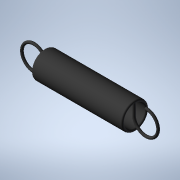
# Autodesk Inventor part: AUA2-10
Saved by Autodesk Inventor 2021 (Build 250183000, 183)
## iProperties
Created: 2025-12-16
Part Number: AUA2-10
Material: Generic
Catalog Web Link: www.3dfindit.com
Description: AWA ,AUA  ,AWY, BWY, AUY, BUY, AWU, BWU, AUU, BUU, AWS, BWS, AUS, BUSS, AWF, AUF,  AWT, BWT, AUT, BUT-Tension Springs - Extralight / Light / Light to Medium / Medium Load / Medium to Heavy / Heavy Load Type
Vendor: MISUMI
Document SubType Name: Modeling
Designer: psAdmin
Manufacturer: MISUMI
Mass: 0.00796164 g
Surface Area: 0.845602 cm^2
Volume: 0.00796164 cm^3
Density: 1 g/cm^3
Appearance: PSOLRGB-176-176-176
Category: PARTsolutions
Company: MISUMI
Title: AUA2-10
Author: Cadenas PARTsolutions
Comments: Tension Springs - Extralight / Light / Light to Medium / Medium Load / Medium to Heavy / Heavy Load Type
PSOL_IDENT_0: {$CADENAS_DATA/23d-libs/misumi/metric/29_springs/awf.prj},261 {VTYP=3D},{NB=AUA2-10},{LINA=AUA2-10},
PSOL_IDENT_1: {NN=AWA ,AUA  ,AWY, BWY, AUY, BUY, AWU, BWU, AUU, BUU, AWS, BWS, AUS, BUSS, AWF, AUF,  AWT, BWT, AUT
PSOL_IDENT_2: , BUT},{DATE=15.09.2021 11:46:20},{GEOMDATE=29.07.2021 01:15:23},{VERSION=},{LINEID=30},{WBVAR=TS,MA
PSOL_IDENT_3: T,TE,L},{WBNUMERIC=L}  {NB=AUA2-10},{LINA=AUA2-10},{KT=DUMMY},{PN=AUA2-10},{TS=5},{TYPE=A},{MAT=U},{
PSOL_IDENT_4: D=2},{TS1='5','Ultra Light Load','1','Light Load','2','Light to Medium Load','3','Medium Load'},{TE=
PSOL_IDENT_5: A},{TE1= 'A','Parallel Ends'},{L=10},{DD=0.20},{L1=10,15,20,25,30},{L5=10,15,20,25,30},{L11=10,15,20
PSOL_IDENT_6: ,25,30},{L2=10,15,20,25},{L22=10,15,20,25},{L3=10,15,20},{L333=10,15,20,25},{L33=10,15,20,25},{L6=0}
PSOL_IDENT_7: ,{L66=0},{L4=0},{L44=0},{LA=10,15,20,25,30},{MD=6.7},{MD1=5.7},{MD2=4},{MD3=3.8},{MD4=0},{MD5=6.7},{
PSOL_IDENT_8: MD6=0.00},{ML=0.69},{IT=0.13},{SC=0.083},{SC1=0.27},{SC2=0.49},{SC3=0.75},{SC4=0},{SC5=0.083},{SC6=0
PSOL_IDENT_9: },{MAT1='W','Spring Steel (ASTM A228)','U','304 Stainless Steel-WPB'},{X=1}
NB: AUA2-10
NN: AWA ,AUA  ,AWY, BWY, AUY, BUY, AWU, BWU, AUU, BUU, AWS, BWS, AUS, BUSS, AWF, AUF,  AWT, BWT, AUT, BUT
NT: Tension Springs - Extralight / Light / Light to Medium / Medium Load / Medium to Heavy / Heavy Load Type
NBSYN: $PN.
LINA: AUA2-10
CATALOG: Misumi
PN: AUA2-10
TS: Ultra Light Load
MAT: 304 Stainless Steel-WPB
D: 2
TE: Parallel Ends
L: 10
DD: 0.2
L66: 0
MD: 6.7
ML: 0.69
IT: 0.13
SC: 0.083
SUPPLIER: MISUMI
ARTICLENO: AUA2-10
BOMINFO: AUA2-10
CREATOR: CADENAS GmbH
Autodesk Inventor part; units mm, degrees
ref_plane "YZ Plane" through (0, 0, 0) normal (1, 0, 0) x (0, 1, 0)
ref_plane "XZ Plane" through (0, 0, 0) normal (0, 1, 0) x (-1, 0, 0)
ref_plane "XY Plane" through (0, 0, 0) normal (0, 0, 1) x (1, 0, 0)
sketch "Sketch_9" plane through (0, 0, 0) normal (0, 0, 1) x (1, 0, 0)
  line L0 (8.4, 0) -> (1.6, 0)
  arc A0 (1.7, 1) -> (1.7, 0.8) centre (1.7, 0.9) ccw
  line L1 (1.7, 0.8) -> (8.3, 0.8)
  arc A1 (8.3, 0.8) -> (8.3, 1) centre (8.3, 0.9) ccw
  line L2 (8.3, 1) -> (1.7, 1)
  constraints: 6 end point, 4 point on circle, 2 centre point
revolve "Revolution1" add sketch "Sketch_9" angle 360 about axis through (8.4, 0, 0) along (1, 0, 0)
sketch "Sketch_10" plane through (0, 0, 0) normal (0, 0, 1) x (1, 0, 0)
  line L0 (8.3, 0) -> (8.3, 0.9)
  line L1 (8.3, 0.9) -> (8.4, 0.9)
  line L2 (8.4, 0.9) -> (8.4, 0)
  line L3 (8.4, 0) -> (8.3, 0)
  line L4 (8.3, 0) -> (8.3, 0.9)
  constraints: 10 end point
revolve "Revolution2" add sketch "Sketch_10" angle 360 about axis through (8.3, 0, 0) along (0, -1, 0)
sketch "Sketch_12" plane through (0, 0, 0) normal (0, 1, 0) x (-1, 0, 0)
  line L0 (-9.2, -1) -> (-9.2, 1)
  circle A0 centre (-8.3, 0) radius 0.1
  constraints: 2 end point, 1 centre point
revolve "Revolution3" add sketch "Sketch_12" angle 271 about axis through (9.2, 0, -1) along (0, 0, 1)
sketch "Sketch_11" plane through (0, 0, 0) normal (0, 0, 1) x (1, 0, 0)
  line L0 (1.7, -0.9) -> (1.7, 0)
  line L1 (1.7, 0) -> (1.8, 0)
  line L2 (1.8, 0) -> (1.8, -0.9)
  line L3 (1.8, -0.9) -> (1.7, -0.9)
  line L4 (1.7, -0.9) -> (1.7, 0)
  constraints: 10 end point
revolve "Revolution4" add sketch "Sketch_11" angle 360 about axis through (1.7, -0.9, 0) along (0, 1, 0)
sketch "Sketch_13" plane through (0, 0, 0) normal (0, 1, 0) x (-1, 0, 0)
  line L0 (-0.8, 1) -> (-0.8, -1)
  circle A0 centre (-1.7, 0) radius 0.1
  constraints: 2 end point, 1 centre point
revolve "Revolution5" add sketch "Sketch_13" angle 271 about axis through (0.8, 0, 1) along (0, 0, 1)
body "Solid1"
